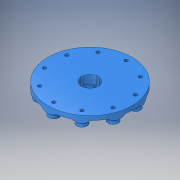
# Autodesk Inventor part: 000.204 - Поворотное основание
Saved by Autodesk Inventor 2019 (Build 230136000, 136)
## iProperties
Created: 2020-03-18
Part Number: 000.204 - Поворотное основание
Material: Пластик АБС
Document SubType Name: Modeling
Designer: Петров Иван
Density: 1.06 g/cm^3
Appearance: Голубой
Author: Петров Иван
Autodesk Inventor part; units mm, degrees
ref_plane "YZ Plane" through (0, 0, 0) normal (1, 0, 0) x (0, 1, 0)
ref_plane "XZ Plane" through (0, 0, 0) normal (0, 1, 0) x (-1, 0, 0)
ref_plane "XY Plane" through (0, 0, 0) normal (0, 0, 1) x (1, 0, 0)
sketch "Эскиз1" plane through (0, 0, 0) normal (0, 1, 0) x (-1, 0, 0)
  circle A0 centre (0, 0) radius 12.425
  dimension "d0" = 24.85
  constraints: 1 centre point, 1 coincident
  measures "d0" diameter of A0
extrude "Выдавливание1" add sketch "Эскиз1" along normal blind 12.7
sketch "Эскиз2" plane through (0, 0, 0) normal (0, -1, 0) x (1, 0, 0)
  circle A0 centre (0, 0) radius 13.8
  circle A1 centre (-8, 0) radius 1.2
  circle A2 centre (0, -8) radius 1.2
  circle A3 centre (8, 0) radius 1.2
  circle A4 centre (0, 8) radius 1.2
  circle A5 centre (-7.7782, 7.7782) radius 1.2813
  circle A6 centre (-11, 0) radius 1.2813
  circle A7 centre (-7.7782, -7.7782) radius 1.2813
  circle A8 centre (0, -11) radius 1.2812
  circle A9 centre (7.7782, -7.7782) radius 1.2812
  circle A10 centre (11, 0) radius 1.2813
  circle A11 centre (7.7782, 7.7782) radius 1.2812
  circle A12 centre (0, 11) radius 1.2812
  circle A13 centre (0, 0) radius 5
  circle A14 centre (0, 0) radius 14
  circle A15 centre (0, 0) radius 1.55
  circle A16 centre (0, 0) radius 1.75
  constraints: 17 centre point
extrude "Выдавливание2" cut sketch "Эскиз2" against normal blind 5 contours A13 | A15 | A16
sketch "Эскиз3" plane through (0, 12.7, 0) normal (0, 1, 0) x (1, 0, 0)
  circle A0 centre (0, 0) radius 23
  dimension "d5" = 46
  constraints: 1 centre point, 1 coincident
  measures "d5" diameter of A0
extrude "Выдавливание3" add sketch "Эскиз3" along normal blind 5 and the other way blind 1
sketch "Эскиз4" plane through (0, 17.7, 0) normal (0, 1, 0) x (1, 0, 0)
  circle A0 centre (0, 0) radius 13.8
  circle A1 centre (-8, 0) radius 1.2
  circle A2 centre (0, -8) radius 1.2
  circle A3 centre (8, 0) radius 1.2
  circle A4 centre (0, 8) radius 1.2
  circle A5 centre (-7.7782, 7.7782) radius 1.2813
  circle A6 centre (-11, 0) radius 1.2813
  circle A7 centre (-7.7782, -7.7782) radius 1.2813
  circle A8 centre (0, -11) radius 1.2812
  circle A9 centre (7.7782, -7.7782) radius 1.2812
  circle A10 centre (11, 0) radius 1.2813
  circle A11 centre (7.7782, 7.7782) radius 1.2812
  circle A12 centre (0, 11) radius 1.2812
  circle A13 centre (0, 0) radius 5
  circle A14 centre (0, 0) radius 14
  circle A15 centre (0, 0) radius 1.55
  circle A16 centre (0, 0) radius 1.75
  constraints: 17 centre point
extrude "Выдавливание4" cut sketch "Эскиз4" against normal through all contours A1 | A2 | A3 | A4 | A15 | A16
sketch "Эскиз5" plane through (0, 17.7, 0) normal (0, 1, 0) x (1, 0, 0)
  circle A0 centre (0, 0) radius 1.75 projected
  circle A1 centre (0, 0) radius 10
  dimension "d12" = 20
  constraints: 1 centre point, 1 coincident
  measures "d12" diameter of A1
extrude "Выдавливание5" cut sketch "Эскиз5" against normal blind 10
sketch "Эскиз6" plane through (0, 17.7, 0) normal (0, 1, 0) x (1, 0, 0)
  circle A0 centre (0, -8) radius 1.2 projected
  circle A1 centre (0, -8) radius 2.5
  point P0 (0, 0)
  dimension "d15" = 5
  constraints: 1 centre point, 1 coincident
  measures "d15" diameter of A1
extrude "Выдавливание6" cut sketch "Эскиз6" against normal blind 15 contours A0 | A1
pattern_circular "Круговой массив1" count 4 over 360 about axis through (0, 17.7, 0) along (0, -1, 0) of "Выдавливание6"
sketch "Эскиз7" plane through (0, 17.7, 0) normal (0, 1, 0) x (1, 0, 0)
  circle A0 centre (0, 0) radius 1.75 projected
  circle A1 centre (0, 0) radius 50
  circle A2 centre (0, 0) radius 23 projected
  arc A3 (9.8594, -1.6711) -> (9.8594, 1.6711) centre (8, 0) ccw projected
  arc A4 (1.6711, -9.8594) -> (9.8594, -1.6711) centre (0, 0) ccw projected
  arc A5 (-1.6711, -9.8594) -> (1.6711, -9.8594) centre (0, -8) ccw projected
  arc A6 (-9.8594, -1.6711) -> (-1.6711, -9.8594) centre (0, 0) ccw projected
  arc A7 (-9.8594, 1.6711) -> (-9.8594, -1.6711) centre (-8, 0) ccw projected
  arc A8 (-1.6711, 9.8594) -> (-9.8594, 1.6711) centre (0, 0) ccw projected
  arc A9 (1.6711, 9.8594) -> (-1.6711, 9.8594) centre (0, 8) ccw projected
  arc A10 (9.8594, 1.6711) -> (1.6711, 9.8594) centre (0, 0) ccw projected
  dimension "d21" = 100
  constraints: 1 centre point, 1 coincident
  measures "d21" diameter of A1
extrude "Выдавливание7" add sketch "Эскиз7" against normal blind 5 contours A1
sketch "Эскиз8" plane through (0, 12.7, 0) normal (0, -1, 0) x (1, 0, 0)
  circle A0 centre (0, 0) radius 1.75 projected
  line L0 (0, 0) -> (0, 43)
  line L1 (0, 47) -> (3.4641, 45)
  line L2 (3.4641, 45) -> (3.4641, 41)
  line L3 (3.4641, 41) -> (0, 39)
  line L4 (0, 39) -> (-3.4641, 41)
  line L5 (-3.4641, 41) -> (-3.4641, 45)
  line L6 (-3.4641, 45) -> (0, 47)
  circle A1 centre (0, 43) radius 6
  dimension "d24" = 43
  dimension "d25" = 8
  dimension "d28" = 12
  constraints: 14 end point, 2 coincident, 1 centre point, 1 vertical, 13 other
  measures "d24" distance of L0.start L0.end
  measures "d25" distance of L3.end L1.start
  measures "d28" diameter of A1
extrude "Выдавливание8" add sketch "Эскиз8" along normal blind 8 contours A1
chamfer "Фаска1" distance 4.5 angle 45 1 edges at (-6, 12.7, 43)
sketch "Эскиз9" plane through (0, 12.7, 0) normal (0, -1, 0) x (1, 0, 0)
  circle A0 centre (0, 0) radius 1.75
  line L0 (0, 0) -> (0, 43)
  line L1 (0, 47) -> (3.4641, 45)
  line L2 (3.4641, 45) -> (3.4641, 41)
  line L3 (3.4641, 41) -> (0, 39)
  line L4 (0, 39) -> (-3.4641, 41)
  line L5 (-3.4641, 41) -> (-3.4641, 45)
  line L6 (-3.4641, 45) -> (0, 47)
  circle A1 centre (0, 43) radius 6
  circle A2 centre (0, 43) radius 2
  dimension "d32" = 43
  dimension "d33" = 8
  dimension "d34" = 12
  dimension "d35" = 4
  constraints: 14 end point, 3 centre point, 3 coincident, 1 vertical, 13 other
  measures "d32" distance of L0.start L0.end
  measures "d33" distance of L3.end L1.start
  measures "d34" diameter of A1
  measures "d35" diameter of A2
extrude "Выдавливание9" cut sketch "Эскиз9" against normal through all contours A2
pattern_circular "Круговой массив2" count 10 over 360 about axis through (0, 17.7, 0) along (0, 1, 0) of "Выдавливание8", "Фаска1", "Выдавливание9"
sketch "Эскиз10" plane through (0, 17.7, 0) normal (0, 1, 0) x (1, 0, 0)
  circle A0 centre (-25.2748, -34.7877) radius 2 projected
  circle A1 centre (-40.8954, -13.2877) radius 2 projected
  circle A2 centre (-40.8954, 13.2877) radius 2 projected
  circle A3 centre (-25.2748, 34.7877) radius 2 projected
  circle A4 centre (0, 43) radius 2 projected
  circle A5 centre (25.2748, 34.7877) radius 2 projected
  circle A6 centre (40.8954, 13.2877) radius 2 projected
  circle A7 centre (40.8954, -13.2877) radius 2 projected
  circle A8 centre (25.2748, -34.7877) radius 2 projected
  circle A9 centre (0, -43) radius 2 projected
  circle A10 centre (0, 0) radius 50 projected
  arc A11 (9.8594, -1.6711) -> (9.8594, 1.6711) centre (8, 0) ccw projected
  arc A12 (1.6711, -9.8594) -> (9.8594, -1.6711) centre (0, 0) ccw projected
  arc A13 (-1.6711, -9.8594) -> (1.6711, -9.8594) centre (0, -8) ccw projected
  arc A14 (-9.8594, -1.6711) -> (-1.6711, -9.8594) centre (0, 0) ccw projected
  arc A15 (-9.8594, 1.6711) -> (-9.8594, -1.6711) centre (-8, 0) ccw projected
  arc A16 (-1.6711, 9.8594) -> (-9.8594, 1.6711) centre (0, 0) ccw projected
  arc A17 (1.6711, 9.8594) -> (-1.6711, 9.8594) centre (0, 8) ccw projected
  arc A18 (9.8594, 1.6711) -> (1.6711, 9.8594) centre (0, 0) ccw projected
